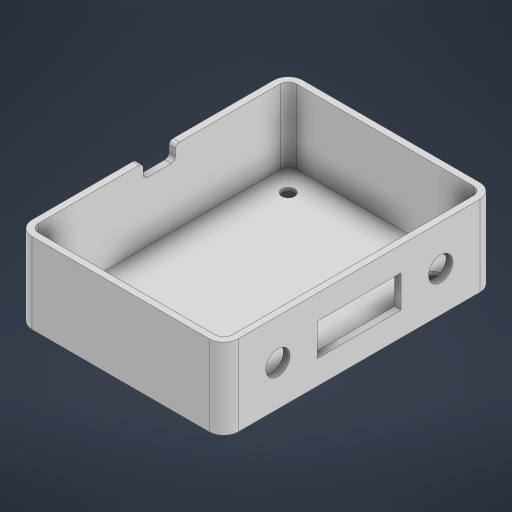
# Autodesk Inventor part: BaseV2
Saved by Autodesk Inventor 2024 (Build 280153000, 153)
## iProperties
Created: 2023-07-31
Part Number: BaseV2
Material: Generic
Document SubType Name: Modeling
Designer: Noah
Density: 1 g/cm^3
Appearance: Default
Author: Noah
## iProperties of the stored document BaseV2_3DPrint.ipt
Created: 2023-07-31
Part Number: BaseV2_3DPrint
Material: Generic
Document SubType Name: Modeling
Designer: Noah
Density: 1 g/cm^3
Appearance: Default
Author: Noah
Autodesk Inventor part; units mm, degrees
ref_plane "YZ Plane" through (0, 0, 0) normal (1, 0, 0) x (0, 1, 0)
ref_plane "XZ Plane" through (0, 0, 0) normal (0, 1, 0) x (-1, 0, 0)
ref_plane "XY Plane" through (0, 0, 0) normal (0, 0, 1) x (1, 0, 0)
sketch "Sketch1" plane through (0, 0, 0) normal (0, 1, 0) x (-1, 0, 0)
  line L0 (0, 0) -> (50, 0)
  line L1 (50, 0) -> (50, -70)
  line L2 (50, -70) -> (0, -70)
  line L3 (0, -70) -> (0, 0)
  line L4 (55, -72.5) -> (55, 2.5)
  line L5 (52.5, 5) -> (-2.5, 5)
  line L6 (-5, 2.5) -> (-5, -72.5)
  line L7 (-2.5, -75) -> (52.5, -75)
  circle A0 centre (47.5, -2.5) radius 2
  line L8 (50, -35) -> (0, -35)
  line L9 (25, 0) -> (25, -70)
  circle A1 centre (47.5, -67.5) radius 2
  circle A2 centre (2.5, -2.5) radius 2
  circle A3 centre (2.5, -67.5) radius 2
  arc A4 (55, 2.5) -> (52.5, 5) centre (52.5, 2.5) ccw
  arc A5 (52.5, -75) -> (55, -72.5) centre (52.5, -72.5) ccw
  arc A6 (-5, -72.5) -> (-2.5, -75) centre (-2.5, -72.5) ccw
  arc A7 (-2.5, 5) -> (-5, 2.5) centre (-2.5, 2.5) ccw
  line L10 (57, 2.5) -> (57, -72.5)
  arc A8 (52.5, -77) -> (57, -72.5) centre (52.5, -72.5) ccw
  line L11 (52.5, -77) -> (-2.5, -77)
  arc A9 (-7, -72.5) -> (-2.5, -77) centre (-2.5, -72.5) ccw
  line L12 (-7, -72.5) -> (-7, 2.5)
  arc A10 (-2.5, 7) -> (-7, 2.5) centre (-2.5, 2.5) ccw
  line L13 (-2.5, 7) -> (52.5, 7)
  arc A11 (57, 2.5) -> (52.5, 7) centre (52.5, 2.5) ccw
  point P0 (25, -35)
  dimension "d0" = 50
  dimension "d1" = 70
  dimension "d2" = 5
  dimension "d3" = 4
  dimension "d4" = 2.5
  dimension "d5" = 2.5
  dimension "d6" = 2.5
  dimension "d7" = 2.5
  dimension "d8" = 2
  constraints: 28 end point, 16 point on circle, 12 centre point, 8 tangent, 6 parallel, 4 midpoint, 3 perpendicular, 3 symmetric about line, 2 equal radius, 1 horizontal, 13 other
  measures "d0" distance of L1.end L2.end
  measures "d1" distance of L0.end L1.end
  measures "d2" distance between parallel lines of L1 L4
  measures "d3" diameter of A0
  measures "d4" distance from line of L0 A0.centre
  measures "d5" distance from line of L1 A0.centre
  measures "d6" radius of A4
  measures "d7" radius of A7
  measures "d8" distance between parallel lines of L4 L10
extrude "Extrusion1" add sketch "Sketch1" along normal blind 2 contours L0 L9 L8 L3 | L0 L1 L8 L9 | L8 L9 L2 L3 | L8 L1 L2 L9 | A5 L7 A6 L6 A7 L5 A4 L4
extrude "Extrusion2" add sketch "Sketch1" along normal blind 25 contours L10 A8 L11 A9 L12 A10 L13 A11
sketch "Sketch2" plane through (0, 0, 0) normal (0, -1, 0) x (1, 0, 0)
  circle A0 centre (-2.5, -2.5) radius 2 projected
  circle A1 centre (-2.5, -2.5) radius 3.5
  circle A2 centre (-47.5, -67.5) radius 2 projected
  circle A3 centre (-47.5, -67.5) radius 3.5
  circle A4 centre (-2.5, -67.5) radius 2 projected
  circle A5 centre (-2.5, -67.5) radius 3.5
  circle A6 centre (-47.5, -2.5) radius 2 projected
  circle A7 centre (-47.5, -2.5) radius 3.5
  point P0 (0, 0)
  dimension "d13" = 7
  dimension "d14" = 7
  dimension "d15" = 7
  dimension "d40" = 7
  constraints: 4 centre point, 4 coincident
  measures "d13" diameter of A3
  measures "d14" diameter of A5
  measures "d15" diameter of A7
  measures "d40" diameter of A1
extrude "Extrusion3" cut sketch "Sketch2" against normal blind 1 contours A0 | A1 | A2 | A3 | A4 | A5 | A6 | A7
sketch "Sketch3" plane through (7, 0, 2.5) normal (1, 0, 0) x (0, 0, -1)
  line L0 (0, 0) -> (75, 0) projected
  line L1 (75, 0) -> (75, 25) projected
  line L2 (0, 25) -> (75, 25) projected
  line L3 (0, 0) -> (0, 25) projected
  line L4 (24.5, 17.5) -> (50.5, 17.5)
  line L5 (50.5, 17.5) -> (50.5, 7.5)
  line L6 (50.5, 7.5) -> (24.5, 7.5)
  line L7 (24.5, 7.5) -> (24.5, 17.5)
  circle A0 centre (12.25, 12.5) radius 3.75
  line L8 (75, 25) -> (0, 25) projected
  line L9 (37.5, 25) -> (37.5, 0)
  circle A1 centre (62.75, 12.5) radius 3.75
  point P0 (2.5, 0)
  point P1 (37.5, 12.5)
  point P2 (37.5, 17.5)
  point P3 (0, 12.5)
  dimension "d18" = 26
  dimension "d19" = 10
  dimension "d20" = 5
  dimension "d21" = 13
  dimension "d22" = 24.5
  dimension "d23" = 24.5
  dimension "d24" = 7.5
  dimension "d25" = 7.5
  dimension "d26" = 7.5
  dimension "d27" = 12.25
  dimension "d28" = 12.25
  dimension "d29" = 12.5
  constraints: 10 end point, 4 midpoint, 2 centre point, 2 parallel, 1 horizontal, 1 perpendicular, 1 symmetric about line, 1 other
  measures "d18" distance of L5.end L6.end
  measures "d19" distance of L4.end L5.end
  measures "d20" distance of point (37.5, 17.5) point (37.5, 12.5)
  measures "d21" distance from line of L7 point (37.5, 12.5)
  measures "d22" distance between parallel lines of L3 L7
  measures "d23" distance between parallel lines of L1 L5
  measures "d24" distance between parallel lines of L0 L6
  measures "d25" distance between parallel lines of L2 L4
  measures "d26" diameter of A0
  measures "d27" distance of point (0, 12.5) A0.centre
  measures "d28" distance from line of L7 A0.centre
  measures "d29" distance from line of L0 A0.centre
extrude "Extrusion4" cut sketch "Sketch3" against normal up to surface (2 mm away) contours L9 L4 L5 L6 | L6 L7 L4 L9 | A0 | A1
sketch "Sketch5" plane through (-57, 0, -72.5) normal (-1, 0, 0) x (0, 0, 1)
  line L0 (32.5, 16) -> (42.5, 16) projected
  line L1 (37.5, 16) -> (37.5, 25)
  line L2 (75, 25) -> (0, 25) projected
  line L3 (37.5, 25) -> (37.5, 20.5)
  line L4 (42.5, 20.5) -> (32.5, 20.5)
  line L5 (32.5, 20.5) -> (32.5, 25)
  line L6 (32.5, 25) -> (42.5, 25)
  line L7 (42.5, 25) -> (42.5, 20.5)
  line L8 (42.5, 20.5) -> (32.5, 25) construction
  line L9 (32.5, 20.5) -> (42.5, 25) construction
  point P0 (72.5, 0)
  point P1 (37.5, 22.75)
  constraints: 16 end point, 6 midpoint, 2 parallel, 1 horizontal, 1 perpendicular, 1 point on line
extrude "Extrusion6" cut sketch "Sketch5" against normal up to surface (2 mm away)
fillet "Fillet1" radius 1.25 4 edges at (-56, 25, -40) (-56, 25, -30) (-56, 20.5, -30) (-56, 20.5, -40)
sketch "Sketch6" plane through (0, 25, 0) normal (0, 1, 0) x (1, 0, 0)
  line L0 (-57, 28.75) -> (-55, 28.75) projected
  line L1 (-57, 28.75) -> (-57, -2.5) projected
  arc A0 (-57, -2.5) -> (-52.5, -7) centre (-52.5, -2.5) ccw projected
  line L2 (-52.5, -7) -> (2.5, -7) projected
  arc A1 (2.5, -7) -> (7, -2.5) centre (2.5, -2.5) ccw projected
  line L3 (7, -2.5) -> (7, 72.5) projected
  arc A2 (7, 72.5) -> (2.5, 77) centre (2.5, 72.5) ccw projected
  line L4 (2.5, 77) -> (-52.5, 77) projected
  arc A3 (-52.5, 77) -> (-57, 72.5) centre (-52.5, 72.5) ccw projected
  line L5 (-57, 72.5) -> (-57, 41.25) projected
  line L6 (-55, 41.25) -> (-57, 41.25) projected
  line L7 (-55, 41.25) -> (-55, 72.5) projected
  arc A4 (-52.5, 75) -> (-55, 72.5) centre (-52.5, 72.5) ccw projected
  line L8 (-52.5, 75) -> (2.5, 75) projected
  arc A5 (5, 72.5) -> (2.5, 75) centre (2.5, 72.5) ccw projected
  line L9 (5, 72.5) -> (5, -2.5) projected
  arc A6 (2.5, -5) -> (5, -2.5) centre (2.5, -2.5) ccw projected
  line L10 (2.5, -5) -> (-52.5, -5) projected
  arc A7 (-55, -2.5) -> (-52.5, -5) centre (-52.5, -2.5) ccw projected
  line L11 (-55, -2.5) -> (-55, 28.75) projected
  point P0 (0, 0)
body "Solid1"
